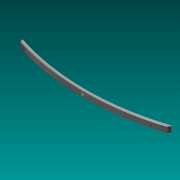
# Autodesk Inventor part: leaf 2
Saved by Autodesk Inventor 2014 SP2 (Build 180246200, 246)
## iProperties
Created: 2019-07-17
Part Number: leaf 2
Material: Steel, Carbon
Document SubType Name: Modeling
Designer: USER PC
Density: 7.87 g/cm^3
Appearance: Semi-Polished
Mass: 2420.37 g
Surface Area: 606.171 cm^2
Volume: 307.544 cm^3
Author: USER PC
Autodesk Inventor part; units mm, degrees
ref_plane "YZ Plane" through (0, 0, 0) normal (1, 0, 0) x (0, 1, 0)
ref_plane "XZ Plane" through (0, 0, 0) normal (0, 1, 0) x (-1, 0, 0)
ref_plane "XY Plane" through (0, 0, 0) normal (0, 0, 1) x (1, 0, 0)
sketch "Sketch1" plane through (0, 0, 0) normal (0, 0, 1) x (1, 0, 0)
  arc A0 (0.4294, -77.1903) -> (350.3978, -24.4313) centre (0.4294, 1109.9183) ccw
  arc A1 (0.2037, -92.1903) -> (354.8199, -38.7647) centre (0.4294, 1109.9183) ccw
  line L0 (0.2076, -71.1704) -> (0.2037, -92.1903)
  line L1 (350.3978, -24.4313) -> (372.3, -24.4313) construction
  line L2 (0, 0) -> (375, 0)
  line L3 (375, 0) -> (375, -16.8411)
  line L4 (350.3978, -24.4313) -> (375, -16.8411)
  line L5 (354.8199, -38.7647) -> (363.9727, -35.9408)
  line L6 (375, -16.8411) -> (363.9727, -35.9408)
  line L7 (375, -16.8411) -> (397.0545, -16.8411) construction
  arc A2 (-349.9649, -24.2998) -> (0.4294, -77.1903) centre (0.4294, 1109.9183) ccw
  arc A3 (-354.3924, -38.6315) -> (0.2037, -92.1903) centre (0.4294, 1109.9183) ccw
  line L8 (-349.9649, -24.2998) -> (-374.5643, -16.7003)
  line L9 (-354.3924, -38.6315) -> (-363.5442, -35.8042)
  line L10 (-374.5643, -16.7003) -> (-363.5442, -35.8042)
  arc A4 (0.4294, -107.1903) -> (359.242, -53.098) centre (0.4294, 1109.9183) ccw
  line L11 (359.242, -53.098) -> (374.0198, -48.5388)
  line L12 (374.0198, -48.5388) -> (388.2749, -23.8483)
  line L13 (363.9727, -35.9408) -> (0.4294, -35.9408)
  point P0 (350.1634, -39.5425)
  point P1 (287.1787, -57.4891)
  dimension "d0" = 15
  dimension "d12" = 375
  dimension "d13" = 120
  dimension "d15" = 15
  dimension "d16" = 363.5433
  constraints: 28 end point, 11 point on circle, 5 centre point, 4 symmetric about line, 3 parallel, 2 horizontal, 2 tangent, 1 equal length, 1 perpendicular, 4 other
  measures "d0" radial gap between concentric circles of A0 A1
  measures "d12" distance of L2.start L2.end
  measures "d13" angle of L6 L7
  measures "d15" radial gap between concentric circles of A4 A1
  measures "d16" distance of L5.end L13.end
extrude "Extrusion1" add sketch "Sketch1" along normal blind 30
sketch "Sketch2" plane through (0, 0, 0) normal (0, 1, 0) x (-1, 0, 0)
  line L0 (0, 0) -> (0, 15)
  circle A0 centre (0, 15) radius 5
  dimension "d5" = 15
  dimension "d6" = 10
  constraints: 2 end point, 1 centre point, 1 coincident, 1 vertical
  measures "d5" distance of L0.start L0.end
  measures "d6" diameter of A0
extrude "Extrusion2" cut sketch "Sketch2" against normal blind 300
fillet "Fillet5" radius 3 17 edges at (359.3963, -37.3527, 30) (-358.9683, -37.2179, 30) (179.5153, -78.7757, 30) (-358.9683, -37.2179, 0) (359.3963, -37.3527, 0) (179.5153, -78.7757, 0) (-363.5442, -35.8042, 15) (-369.0543, -26.2523, 30) (-362.2646, -20.5001, 30) (362.6989, -20.6362, 30) (-176.7524, -63.8932, 30) (-369.0543, -26.2523, 0) (-374.5643, -16.7003, 15) (369.4864, -26.3909, 0) (363.9727, -35.9408, 15) (369.4864, -26.3909, 30) (375, -16.8411, 15)
body "Solid1"
